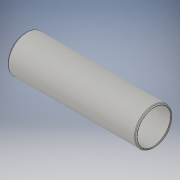
# Autodesk Inventor part: 09R-3.81350SR
Saved by Autodesk Inventor 2016 SP1 (Build 200210100, 210)
## iProperties
Category: PARTsolutions
Company: BIMBA
Created: 2017-03-09
Part Number: 09R-3.81350SR
Material: Generic
Catalog Web Link: www.cadenas.de
Description: Tube-Original Line - Standard Air Cylinders
Vendor: BIMBA
Document SubType Name: Standard Catalog Part
Designer: 589013
Manufacturer: BIMBA
Mass: 4.56811 g
Surface Area: 172.515 cm^2
Volume: 4.56811 cm^3
Density: 1 g/cm^3
Appearance: PSOLRGB-180-180-180
PSOL_IDENT_0: {$CADENAS_DATA\23d-libs\bimba\bimba\bimba_imperial\bimba_full_line\original_line_cylinders\standard_
PSOL_IDENT_1: air_cylinders\tube.prj},194 {VTYP=3D},{NB=09R-3.81350SR},{LINA=09R-3.81350SR},{NN=Tube},{DATE=09.11.
PSOL_IDENT_2: 2016 07:55:11},{GEOMDATE=18.02.2011 00:00:00},{VERSION=},{LINEID=60},{LINESUBID=-1},{WBVAR=MNT,ACTIN
PSOL_IDENT_3: G,NR,L,FOURHOLES,SR}  {NB=09R-3.81350SR},{LINA=09R-3.81350SR},{KT=DUMMY},{PN=09R-3.81350SR},{BORE=1.
PSOL_IDENT_4: 06250000},{BOREPN=09},{MNT=},{MNTALG='' , 'Front Nose' , 'BF' , 'Front Block' , 'BFT' , 'Front Trunn
PSOL_IDENT_5: ion' , 'A' , 'Adjustable Stroke'},{ACTING=R},{ACTINGALG= '' , 'Single Acting' , 'R' , 'Reverse/Doubl
PSOL_IDENT_6: e Acting' },{NR=},{NRALG= '' , 'N/A' },{L=3.8135},{OD=1.1130},{ODN=1.1130},{ODP=1.1130},{ODB=1.1410}
PSOL_IDENT_7: ,{ID=1.0715},{DV=0.00000000},{LV=0.00000000},{LV1=0.00000000},{G=0.0300},{FOURHOLES=0},{AA=0.3750},{
PSOL_IDENT_8: BB=0.0940},{SR=SR},{SRALG= 'C' , 'Carbon Steel Rod' , 'SR' , '303 Stainless Steel Rod' , '' , '303 S
PSOL_IDENT_9: tainless Steel Rod'}
NN: Tube
NT: Original Line - Standard Air Cylinders
NB: 09R-3.81350SR
NBSYN: $PN.
LINA: 09R-3.81350SR
BORE: 1 1/16
BOREPN: 09
MNT: Front Nose
MNTALG: '' , 'Front Nose' , 'BF' , 'Front Block' , 'BFT' , 'Front Trunnion' , 'A' , 'Adjustable Stroke'
ACTING: Reverse/Double Acting
NR: N/A
L: 3.8135
ODN: 1.1130
ODP: 1.1130
ODB: 1.1410
ID: 1.0715
DV: 0.00000000
LV: 0.00000000
LV1: 0.00000000
G: 0.0300
FOURHOLES: 0
AA: 0.3750
BB: 0.0940
SR: 303 Stainless Steel Rod
SUPPLIER: BIMBA
ARTICLENO: 09R-3.81350SR
BOMINFO: 09R-3.81350SR
CREATOR: CADENAS GmbH
Title: 09R-3.81350SR
Author: Cadenas PARTsolutions
Comments: Original Line - Standard Air Cylinders
Autodesk Inventor part; units mm, degrees
sketch "Sketch_1" plane through (0, 0, 0) normal (0, 0, 1) x (1, 0, 0)
  line L0 (96.8629, 0) -> (0, 0)
  arc A0 (-0.6395, 13.2842) -> (-0.6395, 13.1046) centre (-0.5497, 13.1944) ccw
  line L1 (-0.6395, 13.1046) -> (-0.381, 12.846)
  line L2 (-0.381, 12.846) -> (0, 12.846)
  line L3 (0, 12.846) -> (0.762, 13.6081)
  line L4 (0.762, 13.6081) -> (96.1009, 13.6081)
  line L5 (96.1009, 13.6081) -> (96.8629, 12.846)
  line L6 (96.8629, 12.846) -> (97.2439, 12.846)
  line L7 (97.2439, 12.846) -> (97.5024, 13.1046)
  arc A1 (97.5024, 13.1046) -> (97.5024, 13.2842) centre (97.4126, 13.1944) ccw
  line L8 (97.5024, 13.2842) -> (96.8747, 13.9119)
  arc A2 (96.8747, 13.9119) -> (96.3358, 14.1351) centre (96.3359, 13.3731) ccw
  line L9 (96.3358, 14.1351) -> (0.5271, 14.1351)
  arc A3 (0.5271, 14.1351) -> (-0.0118, 13.9119) centre (0.527, 13.3731) ccw
  line L10 (-0.0118, 13.9119) -> (-0.6395, 13.2842)
  constraints: 22 end point, 8 point on circle, 4 centre point
revolve "Revolution1" add sketch "Sketch_1" angle 360 about axis through (96.8629, 0, 0) along (1, 0, 0)
ref_plane "cp1_XY" through (48.4314, 14.1351, 0) normal (1, 0, 0) x (0, 0, -1)
ref_plane "cp1_YZ" through (48.4314, 14.1351, 0) normal (0, 0, -1) x (0, 1, 0)
ref_plane "cp1_ZX" through (48.4314, 14.1351, 0) normal (0, 1, 0) x (1, 0, 0)
ref_plane "cp2_XY" through (48.4314, 0, -14.1351) normal (1, 0, 0) x (0, 0, -1)
ref_plane "cp2_YZ" through (48.4314, 0, -14.1351) normal (0, 0, -1) x (0, 1, 0)
ref_plane "cp2_ZX" through (48.4314, 0, -14.1351) normal (0, 1, 0) x (1, 0, 0)
ref_plane "cp3_XY" through (48.4314, -14.1351, 0) normal (1, 0, 0) x (0, 0, -1)
ref_plane "cp3_YZ" through (48.4314, -14.1351, 0) normal (0, 0, -1) x (0, 1, 0)
ref_plane "cp3_ZX" through (48.4314, -14.1351, 0) normal (0, 1, 0) x (1, 0, 0)
ref_plane "cp4_XY" through (48.4314, 0, 14.1351) normal (1, 0, 0) x (0, 0, -1)
ref_plane "cp4_YZ" through (48.4314, 0, 14.1351) normal (0, 0, -1) x (0, 1, 0)
ref_plane "cp4_ZX" through (48.4314, 0, 14.1351) normal (0, 1, 0) x (1, 0, 0)
ref_plane "tube_front_XY" through (0, 0, 0) normal (1, 0, 0) x (0, 0, -1)
ref_plane "tube_front_YZ" through (0, 0, 0) normal (0, 0, -1) x (0, 1, 0)
ref_plane "tube_front_ZX" through (0, 0, 0) normal (0, 1, 0) x (1, 0, 0)
ref_plane "tube_rear_XY" through (96.8629, 0, 0) normal (1, 0, 0) x (0, 0, -1)
ref_plane "tube_rear_YZ" through (96.8629, 0, 0) normal (0, 0, -1) x (0, 1, 0)
ref_plane "tube_rear_ZX" through (96.8629, 0, 0) normal (0, 1, 0) x (1, 0, 0)
body "Solid1"
